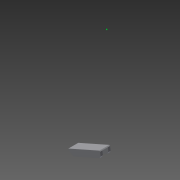
# Autodesk Inventor part: BottomGrip
Saved by Autodesk Inventor 2020.4 (Build 244396010, 396A)
## iProperties
Created: 2022-11-11
Part Number: BottomGrip
Material: Generic
Document SubType Name: Modeling
Designer: Val
Density: 1 g/cm^3
Appearance: Default
Author: Val
Autodesk Inventor part; units mm, degrees
ref_plane "YZ Plane" through (0, 0, 0) normal (1, 0, 0) x (0, 1, 0)
ref_plane "XZ Plane" through (0, 0, 0) normal (0, 1, 0) x (-1, 0, 0)
ref_plane "XY Plane" through (0, 0, 0) normal (0, 0, 1) x (1, 0, 0)
sketch "Sketch1" plane through (0, 0, 0) normal (0, 0, 1) x (1, 0, 0)
  line L0 (-7.3059, -465.3624) -> (-4.6413, -482.4725)
  line L1 (-9.4718, -491.3147) -> (-125.6251, -542.6703)
  line L2 (-125.6251, -542.6703) -> (-148.9715, -527.9978)
  line L3 (-148.9715, -527.9978) -> (-7.3059, -465.3624) construction
  line L4 (-7.3059, -465.3624) -> (-10.4732, -462.5969)
  line L5 (-10.4732, -462.5969) -> (-149.0606, -523.8714)
  line L6 (-149.0606, -523.8714) -> (-148.9715, -527.9978)
  line L7 (-9.4718, -491.3147) -> (-4.6413, -482.4725)
  point P0 (0, 0)
  point P1 (-3.6641, -488.7469)
  dimension "d3" = 3.81
  dimension "d6" = 133.35
  dimension "d8" = 6.35
  dimension "d9" = 6.35
  constraints: 16 end point, 2 point on line
  measures "d3" distance between parallel lines of L5 L3
  measures "d6" distance of point (-3.664, -488.747) L1.end
  measures "d8" distance of L7.start point (-3.664, -488.747)
  measures "d9" distance of L0.end point (-3.664, -488.747)
extrude "Extrusion1" add sketch "Sketch1" along normal mid plane 44.45
sketch "Sketch2" plane through (-138.2759, -548.2636, 22.225) normal (-0.4043748, 0.9145934, 0) x (0.9145934, 0.4043748, 0)
  line L0 (-1.5872, 10) -> (153.3074, 10) construction
  line L1 (153.3074, 34.45) -> (-1.5872, 34.45) construction
  line L2 (163.3576, 10) -> (-32.3991, 10)
  line L3 (-32.3991, 10) -> (-32.3991, 34.45)
  line L4 (-32.3991, 34.45) -> (163.3576, 34.45)
  line L5 (163.3576, 34.45) -> (163.3576, 10)
  line L6 (163.3576, 6.0918) -> (163.3576, 38.3582) construction
  line L7 (-32.3991, 3.3518) -> (-32.3991, 41.0982) construction
  point P0 (348.1702, 22.225)
  constraints: 8 end point, 4 collinear, 2 parallel, 1 horizontal, 1 perpendicular
ref_plane "Work Plane1" through (-188.0551, -545.2781, -26.8885) normal (-0.4043748, 0.9145934, 0) x (0, 0, 1)
extrude "Extrusion2" cut sketch "Sketch2" along normal up to surface (22.86 mm away)
sketch "Sketch4" plane through (0, 0, 0) normal (0, 0, 1) x (1, 0, 0)
  point P0 (0, 0)
equation "\"d9\" = d8"
body "Solid1"
